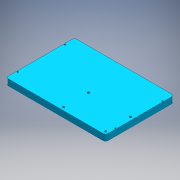
# Autodesk Inventor part: sampleHolderBase_v1
Saved by Autodesk Inventor 2016 (Build 200138000, 138)
## iProperties
Created: 2016-04-12
Part Number: sampleHolderBase_v1
Material: Generic
Document SubType Name: Modeling
Designer: sims01
Density: 1 g/cm^3
Appearance: Default
Author: sims01
Autodesk Inventor part; units mm, degrees
ref_plane "YZ Plane" through (0, 0, 0) normal (1, 0, 0) x (0, 1, 0)
ref_plane "XZ Plane" through (0, 0, 0) normal (0, 1, 0) x (-1, 0, 0)
ref_plane "XY Plane" through (0, 0, 0) normal (0, 0, 1) x (1, 0, 0)
sketch "Sketch1" plane through (0, 0, 0) normal (0, 0, 1) x (1, 0, 0)
  line L0 (-76, 55) -> (76, 55)
  line L1 (80, 51) -> (80, -51)
  line L2 (76, -55) -> (-76, -55)
  line L3 (-80, -51) -> (-80, 51)
  arc A0 (80, 51) -> (76, 55) centre (76, 51) ccw
  arc A1 (76, -55) -> (80, -51) centre (76, -51) ccw
  arc A2 (-76, 55) -> (-80, 51) centre (-76, 51) ccw
  arc A3 (-80, -51) -> (-76, -55) centre (-76, -51) ccw
  point P0 (0, 0)
  point P1 (-80, 55)
  point P2 (80, -55)
  point P3 (80, 55)
  dimension "d0" = 160
  dimension "d1" = 110
  dimension "d2" = 55
  dimension "d3" = 80
  dimension "d4" = 4
  constraints: 8 end point, 8 point on circle, 8 tangent, 6 point on line, 4 centre point, 3 equal radius, 2 parallel, 1 horizontal, 1 perpendicular
  measures "d0" distance of point (-80, 55) point (80, 55)
  measures "d1" distance of point (80, 55) point (80, -55)
  measures "d2" distance from line of point (0, 0) L0
  measures "d3" distance from line of point (0, 0) L1
  measures "d4" radius of A0
extrude "Extrusion1" add sketch "Sketch1" along normal blind 10
sketch "Sketch2" plane through (0, 0, 10) normal (0, 0, 1) x (1, 0, 0)
  point P0 (0, 0)
  point P1 (-78.3, 38)
  point P2 (78.3, 38)
  point P3 (78.3, -38)
  point P4 (-78.3, -38)
  dimension "d7" = 156.6
  dimension "d8" = 76
  dimension "d9" = 38
  dimension "d10" = 78.3
  constraints: 2 horizontal alignment, 2 vertical alignment
  measures "d7" distance of point (78.3, 38) point (-78.3, 38)
  measures "d8" distance of point (-78.3, -38) point (-78.3, 38)
  measures "d9" vertical distance of point (0, 0) point (-78.3, 38)
  measures "d10" horizontal distance of point (0, 0) point (-78.3, 38)
hole "Hole1" at (-78.3, 38, 10) at (78.3, 38, 10) at (78.3, -38, 10) at (-78.3, -38, 10) direction (0, 0, -1) diameter 2.013 end through all thread size "M2.5x0.45" class "6H" standard "ISO Metric profile"
sketch "Sketch3" plane through (0, 0, 10) normal (0, 0, 1) x (1, 0, 0)
  line L0 (-76, -55) -> (76, -55) projected
  line L1 (80, -51) -> (80, 51) projected
  point P0 (0, 0)
  point P1 (7.5, -50)
  point P2 (7.5, -10)
  point P3 (75, -10)
  point P4 (75, -50)
  dimension "d18" = 40
  dimension "d19" = 67.5
  dimension "d20" = 5
  dimension "d21" = 5
  constraints: 2 horizontal alignment, 2 vertical alignment
  measures "d18" distance of point (7.5, -50) point (7.5, -10)
  measures "d19" distance of point (75, -10) point (7.5, -10)
  measures "d20" distance from line of L0 point (7.5, -50)
  measures "d21" distance from line of L1 point (75, -10)
hole "Hole2" at (7.5, -50, 10) at (7.5, -10, 10) at (75, -10, 10) at (75, -50, 10) direction (0, 0, -1) diameter 3.242 end through all thread size "M4x0.7" class "6H" standard "ISO Metric profile"
equation "\"d2\" = 0.5 * d1"
equation "\"d3\" = 0.5 * d0"
equation "\"d9\" = 0.5 * d8"
equation "\"d10\" = 0.5 * d7"
body "Solid1"
